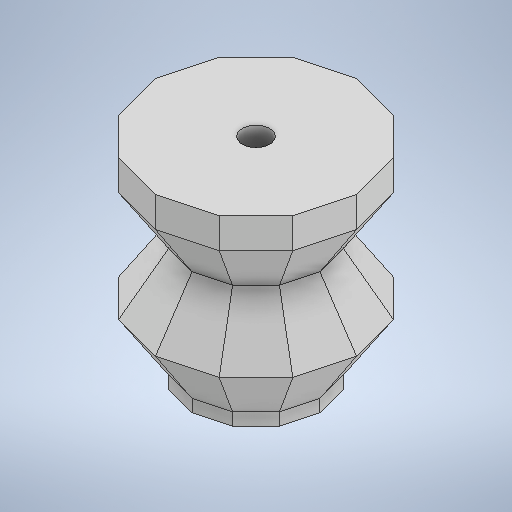
# Autodesk Inventor part: diameter33mm
Saved by Autodesk Inventor 2025.1 (Build 291241000, 241)
## iProperties
Created: 2024-08-09
Part Number: diameter33mm
Material: 일반
Document SubType Name: Modeling
Designer: 82103
Density: 1 g/cm^3
Appearance: 기본값
Author: 82103
Autodesk Inventor part; units mm, degrees
ref_plane "YZ Plane" through (0, 0, 0) normal (1, 0, 0) x (0, 1, 0)
ref_plane "XY Plane" through (0, 0, 0) normal (0, 0, 1) x (1, 0, 0)
sketch "스케치1" plane through (0, 0, 0) normal (0, 1, 0) x (-1, 0, 0)
  line L0 (8.25, -14.2894) -> (0, -16.5)
  line L1 (0, -16.5) -> (-8.25, -14.2894)
  line L2 (-8.25, -14.2894) -> (-14.2894, -8.25)
  line L3 (-14.2894, -8.25) -> (-16.5, 0)
  line L4 (-16.5, 0) -> (-14.2894, 8.25)
  line L5 (-14.2894, 8.25) -> (-8.25, 14.2894)
  line L6 (-8.25, 14.2894) -> (0, 16.5)
  line L7 (0, 16.5) -> (8.25, 14.2894)
  line L8 (8.25, 14.2894) -> (14.2894, 8.25)
  line L9 (14.2894, 8.25) -> (16.5, 0)
  line L10 (16.5, 0) -> (14.2894, -8.25)
  line L11 (14.2894, -8.25) -> (8.25, -14.2894)
  point P0 (0, 0)
  point P1 (0, 0)
  dimension "d0" = 33
  constraints: 24 end point, 1 coincident, 1 horizontal alignment, 25 other
  measures "d0" distance of L3.end L9.end
ref_plane "작업 평면1" through (0, 9, 0) normal (0, 1, 0) x (-1, 0, 0)
sketch "스케치2" plane through (0, 9, 0) normal (0, 1, 0) x (-1, 0, 0)
  line L0 (9.0933, -5.25) -> (5.25, -9.0933)
  line L1 (5.25, -9.0933) -> (0, -10.5)
  line L2 (0, -10.5) -> (-5.25, -9.0933)
  line L3 (-5.25, -9.0933) -> (-9.0933, -5.25)
  line L4 (-9.0933, -5.25) -> (-10.5, 0)
  line L5 (-10.5, 0) -> (-9.0933, 5.25)
  line L6 (-9.0933, 5.25) -> (-5.25, 9.0933)
  line L7 (-5.25, 9.0933) -> (0, 10.5)
  line L8 (0, 10.5) -> (5.25, 9.0933)
  line L9 (5.25, 9.0933) -> (9.0933, 5.25)
  line L10 (9.0933, 5.25) -> (10.5, 0)
  line L11 (10.5, 0) -> (9.0933, -5.25)
  point P0 (0, 0)
  point P1 (0, 0)
  dimension "d2" = 21
  constraints: 24 end point, 1 coincident, 1 horizontal alignment, 25 other
  measures "d2" distance of L4.end L10.end
loft "로프트1" add profiles "스케치2", "스케치1"
mirror "미러1" about plane through (0, 9, 0) normal (0, 1, 0) of "로프트1"
mirror "미러2" about plane through (0, 0, 0) normal (0, 1, 0) of "로프트1"
shell "쉘1" thickness 0.5 removed faces 0 ; own thickness 2 on faces at (-14.4617, -1.5, 3.875) (-10.5867, -1.5, 10.5867) (-3.875, -1.5, 14.4617) (3.875, -1.5, 14.4617) (10.5867, -1.5, 10.5867) (14.4617, -1.5, 3.875) (14.4617, -1.5, -3.875) (10.5867, -1.5, -10.5867) (3.875, -1.5, -14.4617) (-3.875, -1.5, -14.4617) (-10.5867, -1.5, -10.5867) (-14.4617, -1.5, -3.875) (-14.4617, 16.5, -3.875) (-14.4617, 16.5, 3.875) (-10.5867, 16.5, 10.5867) (-3.875, 16.5, 14.4617) (3.875, 16.5, 14.4617) (10.5867, 16.5, 10.5867) (14.4617, 16.5, 3.875) (14.4617, 16.5, -3.875) (10.5867, 16.5, -10.5867) (3.875, 16.5, -14.4617) (-3.875, 16.5, -14.4617) (-10.5867, 16.5, -10.5867)
sketch "스케치3" plane through (-5.25, -9, -9.0933) normal (0, -1, 0) x (0.7071068, 0, 0.7071068)
  line L0 (0, 5.4352) -> (0, 0) projected
  line L1 (0, 0) -> (2.7176, -4.707) projected
  line L2 (2.7176, -4.707) -> (7.4246, -7.4246) projected
  line L3 (7.4246, -7.4246) -> (12.8598, -7.4246) projected
  line L4 (12.8598, -7.4246) -> (17.5668, -4.707) projected
  line L5 (17.5668, -4.707) -> (20.2844, 0) projected
  line L6 (20.2844, 0) -> (20.2844, 5.4352) projected
  line L7 (20.2844, 5.4352) -> (17.5668, 10.1422) projected
  line L8 (17.5668, 10.1422) -> (12.8598, 12.8598) projected
  line L9 (12.8598, 12.8598) -> (7.4246, 12.8598) projected
  line L10 (7.4246, 12.8598) -> (2.7176, 10.1422) projected
  line L11 (2.7176, 10.1422) -> (0, 5.4352) projected
  point P0 (10.1422, 2.7176)
extrude "돌출1" add sketch "스케치3" along normal blind 2
sketch "스케치4" plane through (-14.2894, 18, -8.25) normal (0, 1, 0) x (0.7071068, 0, 0.7071068)
  line L0 (0, 0) -> (0, 8.541) projected
  line L1 (4.2705, -7.3967) -> (0, 0) projected
  line L2 (11.6673, -11.6673) -> (4.2705, -7.3967) projected
  line L3 (20.2083, -11.6673) -> (11.6673, -11.6673) projected
  line L4 (27.605, -7.3967) -> (20.2083, -11.6673) projected
  line L5 (31.8756, 0) -> (27.605, -7.3967) projected
  line L6 (31.8756, 8.541) -> (31.8756, 0) projected
  line L7 (27.605, 15.9378) -> (31.8756, 8.541) projected
  line L8 (20.2083, 20.2083) -> (27.605, 15.9378) projected
  line L9 (11.6673, 20.2083) -> (20.2083, 20.2083) projected
  line L10 (4.2705, 15.9378) -> (11.6673, 20.2083) projected
  line L11 (0, 8.541) -> (4.2705, 15.9378) projected
  point P0 (15.9378, 4.2705)
extrude "돌출2" add sketch "스케치4" along normal blind 5
sketch "스케치5" plane through (-14.2894, 23, -8.25) normal (0, 1, 0) x (0.7071068, 0, -0.7071068)
  circle A0 centre (4.2705, -15.9378) radius 2.25
  dimension "d13" = 4.5
  constraints: 1 centre point, 1 coincident
  measures "d13" diameter of A0
extrude "돌출3" cut sketch "스케치5" against normal blind 5.5
